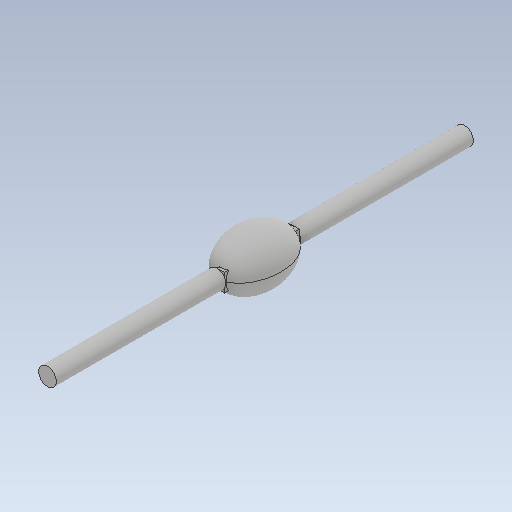
# Autodesk Inventor part: Differential
Saved by Autodesk Inventor 2020 (Build 240168000, 168)
## iProperties
Created: 2020-10-04
Part Number: Differential
Material: Generic
Document SubType Name: Modeling
Designer: nabee
Density: 1 g/cm^3
Appearance: Default
Author: nabee
Autodesk Inventor part; units mm, degrees
ref_plane "YZ Plane" through (0, 0, 0) normal (1, 0, 0) x (0, 1, 0)
sketch "Sketch3" plane through (0, 0, 0) normal (0, 1, 0) x (-1, 0, 0)
  ellipse E0 centre (0, 0) end of major axis (0, 100) minor radius 70.1032
  line L0 (0, 100) -> (0, -100)
  dimension "d6" = 100
  constraints: 2 end point, 1 coincident, 1 vertical, 4 other
revolve "Revolution2" add sketch "Sketch3" angle 360 about axis through (0, 0, 100) along (0, 0, -1) picked at (-23.3548, 1.1091) contours L0 E0
ref_plane "Work Plane2" through (0, 0, -100) normal (0, 0, 1) x (1, 0, 0)
sketch "Sketch4" plane through (0, 0, -100) normal (0, 0, 1) x (1, 0, 0)
  line L0 (70.1032, 0) -> (0, 0) projected
  circle A0 centre (0, 0) radius 23.8125
  dimension "d9" = 47.625
  constraints: 1 centre point, 1 coincident
  measures "d9" diameter of A0
extrude "Extrusion1" add sketch "Sketch4" against normal blind 406.515
ref_plane "Work Plane3" through (0, 0, 100) normal (0, 0, 1) x (1, 0, 0)
sketch "Sketch5" plane through (0, 0, 100) normal (0, 0, 1) x (1, 0, 0)
  line L0 (70.1032, 0) -> (0, 0) projected
  circle A0 centre (0, 0) radius 23.8125
  point P0 (23.8125, 0)
  constraints: 1 centre point, 1 coincident
extrude "Extrusion2" add sketch "Sketch5" along normal blind 406.515
sketch "Sketch6" plane through (0, 0, -506.515) normal (0, 0, -1) x (-1, 0, 0)
  circle A0 centre (0, 0) radius 23.8125
  constraints: 1 centre point, 1 coincident
extrude "Extrusion3" add sketch "Sketch6" along normal blind 46.103
sketch "Sketch7" plane through (0, 0, 506.515) normal (0, 0, 1) x (1, 0, 0)
  circle A0 centre (0, 0) radius 23.8125
  constraints: 1 centre point, 1 coincident
extrude "Extrusion4" add sketch "Sketch7" along normal blind 46.103
sketch "Sketch8" plane through (0, 0, 552.618) normal (0, 0, 1) x (1, 0, 0)
  circle A0 centre (0, 0) radius 23.8125
  constraints: 1 centre point, 1 coincident
extrude "Extrusion5" add sketch "Sketch8" along normal blind 7.794
sketch "Sketch9" plane through (0, 0, 0) normal (1, 0, 0) x (0, 1, 0)
  line L0 (-23.8125, -100) -> (23.8125, -100) projected
  line L1 (-23.8125, 100) -> (23.8125, 100) projected
  line L2 (-23.8125, -100) -> (23.8125, -100)
  line L3 (23.8125, -100) -> (23.8125, 100)
  line L4 (23.8125, 100) -> (-23.8125, 100)
  line L5 (-23.8125, 100) -> (-23.8125, -100)
  point P0 (0, 0)
  constraints: 8 end point, 2 parallel, 1 horizontal, 1 perpendicular
extrude "Extrusion6" add sketch "Sketch9" along normal blind 20
body "Solid2"
